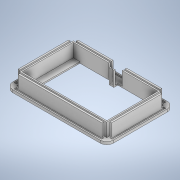
# Autodesk Inventor part: bottom
Saved by Autodesk Inventor 2021 (Build 250183000, 183)
## iProperties
Created: 2021-08-17
Part Number: bottom
Material: Generisch
Document SubType Name: Modeling
Designer: Tilman
Density: 1 g/cm^3
Appearance: Vorgabe
Author: Tilman
Autodesk Inventor part; units mm, degrees
ref_plane "YZ Plane" through (0, 0, 0) normal (1, 0, 0) x (0, 1, 0)
ref_plane "XZ Plane" through (0, 0, 0) normal (0, 1, 0) x (-1, 0, 0)
ref_plane "XY Plane" through (0, 0, 0) normal (0, 0, 1) x (1, 0, 0)
sketch "Skizze1" plane through (0, 0, 0) normal (0, 1, 0) x (-1, 0, 0)
  line L0 (0, 0) -> (-130, 0)
  line L1 (-140, -10) -> (-140, -90)
  line L2 (-130, -100) -> (0, -100)
  line L3 (10, -10) -> (10, -90)
  arc A0 (0, -100) -> (10, -90) centre (0, -90) ccw
  arc A1 (-140, -90) -> (-130, -100) centre (-130, -90) ccw
  arc A2 (-130, 0) -> (-140, -10) centre (-130, -10) ccw
  arc A3 (10, -10) -> (0, 0) centre (0, -10) ccw
  dimension "d0" = 150
  dimension "d1" = 100
  dimension "d2" = 10
  constraints: 8 end point, 8 point on circle, 7 tangent, 4 centre point, 3 equal radius, 2 horizontal, 2 parallel, 2 vertical
  measures "d0" distance between parallel lines of L1 L3
  measures "d1" distance between parallel lines of L0 L2
  measures "d2" radius of A2
extrude "Extrusion1" add sketch "Skizze1" along normal blind 2
sketch "Skizze2" plane through (0, 2, 0) normal (0, 1, 0) x (1, 0, 0)
  line L0 (0, 0) -> (130, 0) projected
  arc A0 (130, 0) -> (140, 10) centre (130, 10) ccw projected
  line L1 (140, 10) -> (140, 90) projected
  arc A1 (140, 90) -> (130, 100) centre (130, 90) ccw projected
  line L2 (130, 100) -> (0, 100) projected
  arc A2 (0, 100) -> (-10, 90) centre (0, 90) ccw projected
  line L3 (-10, 90) -> (-10, 10) projected
  arc A3 (-10, 10) -> (0, 0) centre (0, 10) ccw projected
  line L4 (0, 2) -> (130, 2)
  line L5 (130, 2) -> (130, 5.5)
  line L6 (130, 5.5) -> (0, 5.5)
  line L7 (0, 5.5) -> (0, 2)
  line L8 (138, 10) -> (134.5, 10)
  line L9 (134.5, 10) -> (134.5, 90)
  line L10 (134.5, 90) -> (138, 90)
  line L11 (138, 90) -> (138, 10)
  line L12 (130, 98) -> (0, 98)
  line L13 (0, 98) -> (0, 94.5)
  line L14 (0, 94.5) -> (130, 94.5)
  line L15 (130, 94.5) -> (130, 98)
  line L16 (-8, 90) -> (-4.5, 90)
  line L17 (-4.5, 90) -> (-4.5, 10)
  line L18 (-4.5, 10) -> (-8, 10)
  line L19 (-8, 10) -> (-8, 90)
  line L20 (65, 2) -> (65, 0) construction
  line L21 (0, 0) -> (130, 0) construction
  line L22 (138, 50) -> (140, 50) construction
  line L23 (140, 10) -> (140, 90) construction
  line L24 (65, 98) -> (65, 100) construction
  line L25 (130, 100) -> (0, 100) construction
  line L26 (-8, 50) -> (-10, 50) construction
  line L27 (-10, 90) -> (-10, 10) construction
  line L28 (140, 88) -> (138, 88)
  line L29 (134.5, 88) -> (132.5, 88)
  line L30 (132.5, 88) -> (132.5, 92.5)
  line L31 (132.5, 92.5) -> (128, 92.5)
  line L32 (128, 92.5) -> (128, 94.5)
  line L33 (128, 98) -> (128, 100)
  line L34 (140, 12) -> (138, 12)
  line L35 (134.5, 12) -> (132.5, 12)
  line L36 (132.5, 12) -> (132.5, 7.5)
  line L37 (132.5, 7.5) -> (128, 7.5)
  line L38 (128, 7.5) -> (128, 5.5)
  line L39 (128, 2) -> (128, 0)
  line L40 (2, 0) -> (2, 2)
  line L41 (2, 5.5) -> (2, 7.5)
  line L42 (2, 7.5) -> (-2.5, 7.5)
  line L43 (-2.5, 7.5) -> (-2.5, 12)
  line L44 (-2.5, 12) -> (-4.5, 12)
  line L45 (-8, 12) -> (-10, 12)
  line L46 (-10, 88) -> (-8, 88)
  line L47 (-4.5, 88) -> (-2.5, 88)
  line L48 (-2.5, 88) -> (-2.5, 92.5)
  line L49 (-2.5, 92.5) -> (2, 92.5)
  line L50 (2, 92.5) -> (2, 94.5)
  line L51 (2, 98) -> (2, 100)
  line L52 (-2, 92) -> (132, 92)
  line L53 (132, 92) -> (132, 8)
  line L54 (132, 8) -> (-2, 8)
  line L55 (-2, 8) -> (-2, 92)
  line L56 (130, 90) -> (0, 90)
  line L57 (0, 90) -> (0, 10)
  line L58 (0, 10) -> (130, 10)
  line L59 (130, 10) -> (130, 90)
  line L60 (-2.5, 92.5) -> (0, 90) construction
  line L61 (132.5, 92.5) -> (130, 90) construction
  line L62 (132.5, 7.5) -> (130, 10) construction
  line L63 (-2.5, 7.5) -> (0, 10) construction
  line L64 (2, 88) -> (128, 88)
  line L65 (128, 88) -> (128, 12)
  line L66 (128, 12) -> (2, 12)
  line L67 (2, 12) -> (2, 88)
  line L68 (132.5, 12) -> (132, 12)
  line L69 (128, 7.5) -> (128, 8)
  line L70 (132.5, 88) -> (132, 88)
  line L71 (128, 92.5) -> (128, 92)
  line L72 (2, 92.5) -> (2, 92)
  line L73 (-2.5, 88) -> (-2, 88)
  line L74 (2, 7.5) -> (2, 8)
  line L75 (-2.5, 12) -> (-2, 12)
  point P0 (130, 3.75)
  point P1 (128, 0)
  dimension "d5" = 3.5
  dimension "d6" = 2
  dimension "d7" = 2
  dimension "d12" = 2
  dimension "d13" = 2
  dimension "d14" = 0.5
  dimension "d15" = 2
  constraints: 136 end point, 54 point on line, 25 perpendicular, 20 equal length, 15 parallel, 9 midpoint, 7 horizontal alignment, 7 vertical alignment, 6 horizontal, 3 vertical, 6 other
  measures "d5" distance of L12.end L13.end
  measures "d6" distance of L24.start L24.end
  measures "d7" distance of L49.end L50.end
  measures "d12" distance between parallel lines of L13 L50
  measures "d13" distance between parallel lines of L52 L56
  measures "d14" distance between parallel lines of L48 L55
  measures "d15" distance between parallel lines of L56 L64
extrude "Extrusion2" add sketch "Skizze2" along normal blind 2 contours A3 L3 L45 L19 L18 L17 L44 L43 L42 L41 L6 L7 L4 L40 L0 | L40 L4 L39 L0 | L39 L4 L5 L6 L38 L37 L36 L35 L9 L8 L11 L34 L1 A0 L0 | L3 L46 L19 L45 | L3 A2 L2 L51 L12 L13 L14 L50 L49 L48 L47 L17 L16 L19 L46 | L34 L11 L28 L1 | L28 L11 L10 L9 L29 L30 L31 L32 L14 L15 L12 L33 L2 A1 L1 | L2 L33 L12 L51
extrude "Extrusion4" add sketch "Skizze2" along normal blind 20 contours L41 L74 L54 L69 L38 L6 | L42 L43 L75 L55 L54 L74 | L17 L47 L73 L55 L75 L44 | L69 L54 L53 L68 L36 L37 | L48 L49 L72 L52 L55 L73 | L35 L68 L53 L70 L29 L9 | L14 L32 L71 L52 L72 L50 | L70 L53 L52 L71 L31 L30 | L59 L58 L57 L56
sketch "Skizze3" plane through (0, 22, 0) normal (0, 1, 0) x (1, 0, 0)
  line L0 (132.5, 7.5) -> (132.5, 12) projected
  line L1 (132.5, 12) -> (134.5, 12) projected
  line L2 (134.5, 12) -> (134.5, 88) projected
  line L3 (134.5, 88) -> (132.5, 88) projected
  line L4 (132.5, 88) -> (132.5, 92.5) projected
  line L5 (132.5, 92.5) -> (128, 92.5) projected
  line L6 (128, 92.5) -> (128, 94.5) projected
  line L7 (128, 94.5) -> (2, 94.5) projected
  line L8 (2, 94.5) -> (2, 92.5) projected
  line L9 (2, 92.5) -> (-2.5, 92.5) projected
  line L10 (-2.5, 92.5) -> (-2.5, 88) projected
  line L11 (-2.5, 88) -> (-4.5, 88) projected
  line L12 (-4.5, 88) -> (-4.5, 12) projected
  line L13 (-4.5, 12) -> (-2.5, 12) projected
  line L14 (-2.5, 12) -> (-2.5, 7.5) projected
  line L15 (-2.5, 7.5) -> (2, 7.5) projected
  line L16 (2, 7.5) -> (2, 5.5) projected
  line L17 (2, 5.5) -> (128, 5.5) projected
  line L18 (128, 5.5) -> (128, 7.5) projected
  line L19 (128, 7.5) -> (132.5, 7.5) projected
  line L20 (132, 8) -> (-2, 8) projected
  line L21 (-2, 8) -> (-2, 92) projected
  line L22 (-2, 92) -> (132, 92) projected
  line L23 (132, 92) -> (132, 8) projected
  line L24 (132, 12.5) -> (132, 8)
  line L25 (132, 8) -> (127.5, 8)
  line L26 (127.5, 8) -> (127.5, 6)
  line L27 (127.5, 6) -> (2.5, 6)
  line L28 (2.5, 6) -> (2.5, 8)
  line L29 (2.5, 8) -> (-2, 8)
  line L30 (-2, 8) -> (-2, 12.5)
  line L31 (-2, 12.5) -> (-4, 12.5)
  line L32 (-4, 12.5) -> (-4, 87.5)
  line L33 (-4, 87.5) -> (-2, 87.5)
  line L34 (-2, 87.5) -> (-2, 92)
  line L35 (-2, 92) -> (2.5, 92)
  line L36 (2.5, 92) -> (2.5, 94)
  line L37 (2.5, 94) -> (127.5, 94)
  line L38 (127.5, 94) -> (127.5, 92)
  line L39 (127.5, 92) -> (132, 92)
  line L40 (132, 92) -> (132, 87.5)
  line L41 (132, 87.5) -> (134, 87.5)
  line L42 (134, 87.5) -> (134, 12.5)
  line L43 (134, 12.5) -> (132, 12.5)
  line L44 (2.5, 6) -> (2.5, 5.5)
  line L45 (-4, 12.5) -> (-4.5, 12.5)
  line L46 (-4.5, 10) -> (-4.5, 90) projected
  line L47 (-4, 87.5) -> (-4.5, 87.5)
  line L48 (2.5, 94) -> (2.5, 94.5)
  line L49 (0, 94.5) -> (130, 94.5) projected
  line L50 (127.5, 94) -> (127.5, 94.5)
  line L51 (134, 87.5) -> (134.5, 87.5)
  line L52 (134, 12.5) -> (134.5, 12.5)
  line L53 (127.5, 6) -> (127.5, 5.5)
  line L54 (2, 5.5) -> (128, 5.5) projected
  point P0 (0, 0)
  dimension "d22" = 0.5
  constraints: 56 end point, 12 point on line, 3 perpendicular, 1 parallel, 19 other
  measures "d22" distance between parallel lines of L0 L24
extrude "Extrusion5" cut sketch "Skizze3" against normal up to surface (18 mm away) contours L19 L18 L17 L53 L26 L20 L23 L43 L52 L2 L1 L0 | L51 L41 L23 L22 L38 L50 L7 L6 L5 L4 L3 L2 | L17 L16 L15 L14 L13 L12 L45 L31 L21 L20 L28 L44 | L22 L21 L33 L47 L12 L11 L10 L9 L8 L7 L48 L36
sketch "Skizze4" plane through (0, 2, 0) normal (0, 1, 0) x (1, 0, 0)
  line L0 (2, 88) -> (2, 12) projected
  line L1 (2, 12) -> (128, 12) projected
  line L2 (128, 12) -> (128, 88) projected
  line L3 (128, 88) -> (2, 88) projected
  line L4 (128, 88) -> (2, 88) projected
  line L5 (128, 12) -> (2, 12) projected
  line L6 (12, 88) -> (118, 88)
  line L7 (118, 88) -> (118, 12)
  line L8 (118, 12) -> (12, 12)
  line L9 (12, 12) -> (12, 88)
  line L10 (2, 88) -> (128, 88) projected
  point P0 (0, 0)
  point P1 (65, 88)
  point P2 (12, 12)
  point P3 (118, 12)
  point P4 (118, 88)
  dimension "d25" = 10
  constraints: 8 end point, 2 midpoint, 2 parallel, 2 point on line, 1 horizontal, 1 perpendicular
  measures "d25" distance between parallel lines of L0 L9
extrude "Extrusion6" cut sketch "Skizze4" against normal through all contours L3 L7 L1 L9
sketch "Skizze6" plane through (130, 2, -94.5) normal (0, 0, -1) x (-1, 0, 0)
  line L0 (130, 2) -> (127.5, 2) projected
  line L1 (127.5, 2) -> (127.5, 20) projected
  line L2 (2.5, 20) -> (127.5, 20) projected
  line L3 (2.5, 20) -> (2.5, 2) projected
  line L4 (0, 2) -> (2.5, 2) projected
  line L5 (0, 0) -> (0, 2) projected
  line L6 (130, 0) -> (0, 0) projected
  line L7 (130, 0) -> (130, 2) projected
  line L8 (128, 20) -> (2, 20) projected
  line L9 (55, 20) -> (75, 20)
  line L10 (75, 20) -> (75, 0)
  line L11 (75, 0) -> (55, 0)
  line L12 (55, 0) -> (55, 20)
  point P0 (130, -2)
  point P1 (65, 20)
  point P2 (55, 20)
  point P3 (55, 0)
  point P4 (75, 20)
  dimension "d31" = 20
  constraints: 8 end point, 2 midpoint, 2 parallel, 2 point on line, 1 horizontal, 1 perpendicular
  measures "d31" distance between parallel lines of L10 L12
extrude "Extrusion8" cut sketch "Skizze6" against normal up to surface (6.5 mm away) contours L6 L12 L2 L10
sketch "Skizze7" plane through (0, 0, 0) normal (0, -1, 0) x (1, 0, 0)
  line L0 (118, -12) -> (118, -88) projected
  line L1 (118, -88) -> (12, -88) projected
  line L2 (12, -88) -> (12, -12) projected
  line L3 (12, -12) -> (118, -12) projected
  line L4 (0, 0) -> (130, 0) projected
  arc A0 (0, 0) -> (-10, -10) centre (0, -10) ccw projected
  line L5 (-10, -90) -> (-10, -10) projected
  arc A1 (-10, -90) -> (0, -100) centre (0, -90) ccw projected
  line L6 (130, -100) -> (0, -100) projected
  arc A2 (130, -100) -> (140, -90) centre (130, -90) ccw projected
  line L7 (140, -10) -> (140, -90) projected
  arc A3 (140, -10) -> (130, 0) centre (130, -10) ccw projected
  line L8 (118, -88) -> (12, -88) projected
  line L9 (68.5, -88) -> (61.5, -88)
  line L10 (61.5, -88) -> (61.5, -82)
  line L11 (61.5, -82) -> (68.5, -82)
  line L12 (68.5, -82) -> (68.5, -88)
  line L13 (61.5, -82) -> (63.5, -82)
  line L14 (63.5, -82) -> (63.5, -84)
  line L15 (63.5, -84) -> (61.5, -84)
  line L16 (61.5, -84) -> (61.5, -82)
  line L17 (68.5, -82) -> (66.5, -82)
  line L18 (66.5, -82) -> (66.5, -84)
  line L19 (66.5, -84) -> (68.5, -84)
  line L20 (68.5, -84) -> (68.5, -82)
  point P0 (65, -88)
  point P1 (61.5, -84)
  dimension "d39" = 6
  dimension "d40" = 7
  dimension "d41" = 2
  constraints: 24 end point, 6 parallel, 5 perpendicular, 3 horizontal, 2 midpoint, 2 point on line
  measures "d39" distance of L11.end L9.start
  measures "d40" distance of L10.end L11.end
  measures "d41" distance of L13.end L14.end
extrude "Extrusion9" add sketch "Skizze7" against normal up to surface (22 mm away) contours L19 L18 L11 L12 | L10 L11 L14 L15
extrude "Extrusion10" add sketch "Skizze7" against normal blind 2 contours L1 L10 L15 L14 L11 L18 L19 L12
